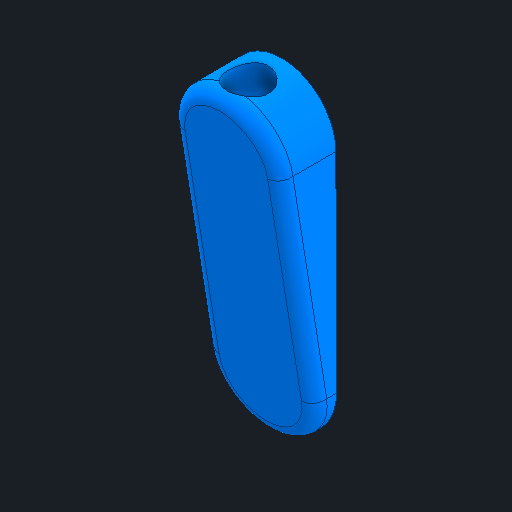
# Autodesk Inventor part: shaft_outlet
Saved by Autodesk Inventor 2023 (Build 270158030, 158C)
## iProperties
Created: 2022-03-28
Part Number: shaft_outlet
Material: Generic
Document SubType Name: Modeling
Designer: kardo
Density: 1 g/cm^3
Appearance: Blue Plastic
Author: kardo
Autodesk Inventor part; units mm, degrees
ref_plane "YZ Plane" through (0, 0, 0) normal (1, 0, 0) x (0, 1, 0)
ref_plane "XZ Plane" through (0, 0, 0) normal (0, 1, 0) x (-1, 0, 0)
ref_plane "XY Plane" through (0, 0, 0) normal (0, 0, 1) x (1, 0, 0)
derived "stencil_frame.ipt"
sketch "sk_drivetrain_profile" plane through (6, 0, 0) normal (1, 0, 0) x (0, 1, 0)
  line L0 (-547.3485, 0) -> (393.091, 0) construction
  line L1 (-363, 4666.1952) -> (-363, -2045.0469) construction
  line L2 (0, 4666.1952) -> (0, -2045.0469) construction
  line L3 (-140.6277, 54.4571) -> (-133.8539, 27.2888)
  line L4 (-388, 0) -> (-343.0839, 2.7472)
  line L5 (-137.2408, 40.8729) -> (-226.9463, 18.5069)
  line L6 (-320.2745, 4.1423) -> (-272.9504, 7.0367) construction
  line L7 (-272.9504, 7.0367) -> (-226.9463, 18.5069) construction
  line L8 (-133.8539, 27.2888) -> (-133.8539, 22.2888) construction
  line L9 (-343.0839, 2.7472) -> (-320.2745, 4.1423)
  line L10 (-1246.9714, 4491.7596) -> (383.4376, -2047.4538) construction
  spline S0 degree 2 poles (-320.2745, 4.1423) (-272.9504, 7.0367) (-226.9463, 18.5069) knots 1 1 1 2 2 2
  line L11 (-227.5223, 20.8174) -> (-137.8168, 43.1835) construction
  line L12 (-136.6647, 38.5624) -> (-226.3702, 16.1963) construction
  line L13 (-227.5223, 20.8174) -> (-226.3702, 16.1963) construction
  line L14 (0, 21.4767) -> (-254.1001, 20.7404) construction
  line L15 (-55.6943, 22.5153) -> (-309.842, 21.7788) construction
  point P0 (0, 0)
  point P1 (-217.5636, 20.8462)
  point P2 (-207.6048, 20.8751)
  point P3 (-202.7352, 22.0892)
sketch "sk_prop_shaft_cut" plane through (6, 0, 21.4767) normal (0, -0.0028978, 0.9999958) x (0, -0.9999958, -0.0028978)
  line L0 (227.5233, -4.3812) -> (202.7326, -4.3812)
  line L1 (227.5233, 4.3812) -> (202.7326, 4.3812)
  arc A0 (202.7326, 4.3812) -> (202.7326, -4.3812) centre (202.7326, 0) ccw
  arc A1 (227.5233, -4.3812) -> (227.5233, 4.3812) centre (227.5233, 0) ccw
  point P0 (0.0622, -6)
  point P1 (217.5645, 0)
  point P2 (207.6056, 0)
ref_plane "plane_motor_mount" through (0, -127.05, 0) normal (0, 0.9702957, 0.2419219) x (-1, 0, 0)
derived "parameters_powertrain.ipt"
derived "parameters_frame.ipt"
extrude "lower_plate" add sketch "sk_prop_shaft_cut" along normal blind 1.2
sketch "sk_upper_plate" plane through (6, -227.5258, 22.0174) normal (0, -0.0028978, 0.9999958) x (1, 0, 0)
  line L0 (-4.3812, 24.7907) -> (-4.3812, 0) projected
  arc A0 (-4.3812, 0) -> (4.3812, 0) centre (0, 0) ccw projected
  line L1 (4.3812, 0) -> (4.3812, 24.7907) projected
  arc A1 (4.3812, 24.7907) -> (-4.3812, 24.7907) centre (0, 24.7907) ccw projected
  line L2 (-6.3812, 0) -> (-6.3813, 24.7907)
  arc A2 (6.3812, 24.7907) -> (-6.3813, 24.7907) centre (0, 24.7907) ccw
  line L3 (6.3812, 24.7907) -> (6.3812, 0)
  arc A3 (-6.3812, 0) -> (6.3812, 0) centre (0, 0) ccw
  point P0 (-6, 227.4611)
  dimension "d6" = 2
  constraints: 4 end point, 4 point on circle, 2 centre point, 3 other
  measures "d6" distance between parallel lines of L2 L0
extrude "upper_plate" add sketch "sk_upper_plate" along normal blind 7.62 contours A1 L1 A0 L0 | L2 A2 L3 A3
sketch "sk_trim" plane through (12.3812, -227.5258, 22.0174) normal (1, 0, 0) x (0, 0.0028978, -0.9999958)
  line L0 (-1.6669, -6.3813) -> (-7.62, 31.172)
  line L1 (0, 0) -> (0, -6.3812) projected
  line L2 (-7.62, 31.172) -> (-7.62, 24.7907) projected
  line L3 (0, -6.3812) -> (-1.6669, -6.3813)
  line L4 (-1.6669, -6.3813) -> (-7.62, -6.3813)
  line L5 (-7.62, -6.3813) -> (-7.62, 24.7907)
  dimension "d16" = 1.6669
  constraints: 8 end point, 2 collinear, 1 perpendicular
  measures "d16" distance of L1.end L0.start
extrude "trim" cut sketch "sk_trim" against normal through all
sketch "sk_drill" plane through (0, -127.05, 0) normal (0, 0.9702957, 0.2419219) x (-1, 0, 0)
  circle A0 centre (-6, 42.1242) radius 2.3813
  point P0 (0, -30.7362)
  dimension "d9" = 4.7625
  constraints: 1 centre point, 1 coincident
  measures "d9" diameter of A0
extrude "drill" cut sketch "sk_drill" along normal through all both and the other way through all
fillet "Fillet1" radius 1.5 6 edges at (10.5122, -232.0437, 23.9674) (1.4878, -232.0437, 23.9674) (-0.3812, -215.144, 26.6967) (10.5122, -198.2442, 29.426) (1.4878, -198.2442, 29.426) (12.3813, -215.144, 26.6967)
equation "\"d4\" = shell_thickness"
equation "\"d7\" = 1.6 * prop_shaft_od"
equation "\"d16\" = 0.35 * prop_shaft_od"
equation "\"d9\" = prop_shaft_od"
equation "\"shell_thickness\" = 1.2"
equation "\"prop_shaft_od\" = 4.7625"
body "Solid1"
